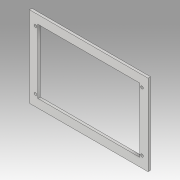
# Autodesk Inventor part: top_instrumentboard
Saved by Autodesk Inventor 2019.3 (Build 233278000, 278)
## iProperties
Created: 2019-05-28
Part Number: top_instrumentboard
Material: Generic
Document SubType Name: Modeling
Designer: Dave
Density: 1 g/cm^3
Appearance: Default
Author: Dave
Autodesk Inventor part; units mm, degrees
ref_plane "YZ Plane" through (0, 0, 0) normal (1, 0, 0) x (0, 1, 0)
ref_plane "XZ Plane" through (0, 0, 0) normal (0, 1, 0) x (-1, 0, 0)
ref_plane "XY Plane" through (0, 0, 0) normal (0, 0, 1) x (1, 0, 0)
sketch "Sketch1" plane through (0, 0, 0) normal (0, 0, 1) x (1, 0, 0)
  line L0 (0, 0) -> (142, 0)
  line L1 (142, 0) -> (142, 97)
  line L2 (142, 97) -> (0, 97)
  line L3 (0, 97) -> (0, 0)
  line L4 (10, 87) -> (132, 87)
  line L5 (132, 87) -> (132, 10)
  line L6 (132, 10) -> (10, 10)
  line L7 (10, 10) -> (10, 87)
  circle A0 centre (7.2, 83.8) radius 1.55
  circle A1 centre (7.2, 13.2) radius 1.55
  circle A2 centre (134.8, 83.8) radius 1.55
  circle A3 centre (134.8, 13.2) radius 1.55
  point P0 (71, 87)
  dimension "d0" = 122
  dimension "d1" = 77
  dimension "d2" = 10
  dimension "d3" = 10
  dimension "d4" = 10
  dimension "d5" = 10
  dimension "d6" = 3.1
  dimension "d7" = 127.6
  dimension "d8" = 63.8
  dimension "d9" = 70.6
  dimension "d10" = 3.2
  dimension "d11" = 3.2
  constraints: 16 end point, 4 centre point, 4 parallel, 3 equal radius, 2 horizontal, 2 horizontal alignment, 2 perpendicular, 2 vertical alignment, 1 midpoint
  measures "d0" distance of L4.start L4.end
  measures "d1" distance of L4.end L5.end
  measures "d2" distance between parallel lines of L7 L3
  measures "d3" distance between parallel lines of L1 L5
  measures "d4" distance between parallel lines of L2 L4
  measures "d5" distance between parallel lines of L6 L0
  measures "d6" diameter of A0
  measures "d7" distance of A2.centre A0.centre
  measures "d8" horizontal distance of A0.centre point (71, 87)
  measures "d9" distance of A3.centre A2.centre
  measures "d10" distance from line of L4 A0.centre
  measures "d11" distance from line of L6 A1.centre
extrude "Extrusion1" add sketch "Sketch1" along normal blind 3
body "Solid1"
